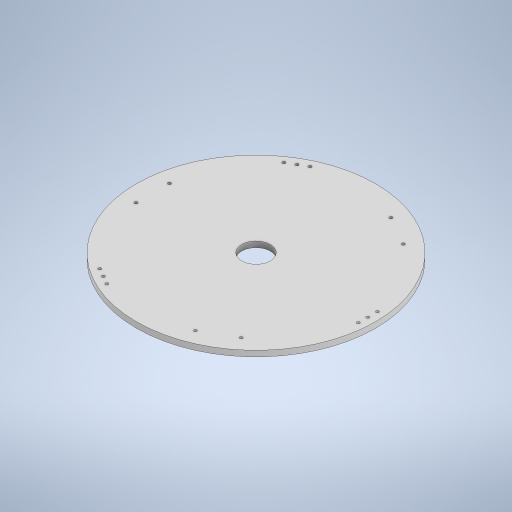
# Autodesk Inventor part: 底板
Saved by Autodesk Inventor 2023 (Build 270158000, 158)
## iProperties
Created: 2022-10-20
Part Number: 底板
Material: 一般
Document SubType Name: Modeling
Designer: Kuri1
Density: 1 g/cm^3
Appearance: 既定
Author: Kuri1
Autodesk Inventor part; units mm, degrees
ref_plane "YZ Plane" through (0, 0, 0) normal (1, 0, 0) x (0, 1, 0)
ref_plane "XZ Plane" through (0, 0, 0) normal (0, 1, 0) x (-1, 0, 0)
ref_plane "XY Plane" through (0, 0, 0) normal (0, 0, 1) x (1, 0, 0)
sketch "スケッチ1" plane through (0, 0, 0) normal (0, 1, 0) x (-1, 0, 0)
  circle A0 centre (0, 0) radius 125
  dimension "d0" = 250
  constraints: 1 centre point, 1 coincident
  measures "d0" diameter of A0
sketch "スケッチ2" plane through (0, 0, 0) normal (0, 1, 0) x (-1, 0, 0)
  circle A0 centre (108, 17.5) radius 1.6
  circle A1 centre (108, -17.5) radius 1.6
  circle A2 centre (-38.8446, 102.2807) radius 1.6
  circle A3 centre (-69.1554, 84.7807) radius 1.6
  circle A4 centre (-69.1554, -84.7807) radius 1.6
  circle A5 centre (-38.8446, -102.2807) radius 1.6
  point P0 (0, 0)
  dimension "d5" = 3.2
  dimension "d6" = 3.2
  dimension "d11" = 35
  dimension "d16" = 360
  dimension "d22" = 108
  dimension "d23" = 108
  dimension "d28" = 17.5
  constraints: 6 centre point, 13 other
  measures "d5" diameter of A0
  measures "d6" diameter of A1
  measures "d11" distance of A0.centre A1.centre
  measures "d22" horizontal distance of point (0, 0) A0.centre
  measures "d23" horizontal distance of point (0, 0) A1.centre
  measures "d28" vertical distance of point (0, 0) A1.centre
extrude "押し出し5" add sketch "スケッチ1" against normal blind 6
extrude "押し出し6" cut sketch "スケッチ2" against normal blind 6
sketch "スケッチ4" plane through (0, 0, 0) normal (0, 1, 0) x (1, 0, 0)
  circle A0 centre (0, 0) radius 116.86
  line L0 (0, 0) -> (-58.43, 101.2037)
  line L1 (0, 0) -> (116.86, 0) construction
  line L2 (0, 0) -> (-58.43, -101.2037)
  line L3 (0, 0) -> (116.86, 0) construction
  line L4 (0, 0) -> (116.86, 0)
  dimension "d33" = 233.72
  dimension "d34" = 120
  dimension "d35" = 120
  constraints: 10 end point, 4 coincident, 3 horizontal, 2 equal length, 2 point on circle, 1 centre point
  measures "d33" diameter of A0
  measures "d34" angle of L1 L0
  measures "d35" angle of L2 L3
hole "穴1" at (-58.43, 0, -101.2037) at (-58.43, 0, 101.2037) at (116.86, 0, 0) direction (0, -1, 0) diameter 3.2 depth 10
sketch "スケッチ5" plane through (0, 0, 0) normal (0, 1, 0) x (1, 0, 0)
  circle A0 centre (116.86, 0) radius 1.6 projected
  line L0 (116.86, 0) -> (116.86, 10)
  line L1 (116.86, 0) -> (126.86, 0) construction
  line L2 (116.86, 10) -> (116.86, -10)
  point P0 (0, 0)
  point P1 (-67.0903, 96.2037)
  point P2 (-49.7697, 106.2037)
  point P3 (-49.7697, -106.2037)
  point P4 (-67.0903, -96.2037)
  dimension "d43" = 10
  dimension "d44" = 90
  dimension "d45" = 20
  dimension "d48" = 360
  constraints: 6 end point, 2 coincident, 1 horizontal, 1 perpendicular, 1 point on line, 1 vertical, 7 other
  measures "d43" distance of L0.start L0.end
  measures "d44" angle of L1 L0
  measures "d45" distance of L0.end L2.end
hole "穴2" at (116.86, 0, -10) at (116.86, 0, 10) at (-67.0903, 0, -96.2037) at (-49.7697, 0, -106.2037) at (-49.7697, 0, 106.2037) at (-67.0903, 0, 96.2037) direction (0, -1, 0) diameter 3.2 depth 10
sketch "スケッチ6" plane through (0, 0, 0) normal (0, 1, 0) x (1, 0, 0)
  circle A0 centre (0, 0) radius 15
  dimension "d57" = 30
  constraints: 1 centre point, 1 coincident
  measures "d57" diameter of A0
extrude "押し出し7" cut sketch "スケッチ6" against normal blind 10
